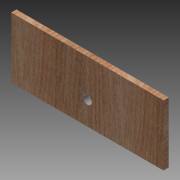
# Autodesk Inventor part: CNC-X-axis- foundation faces
Saved by Autodesk Inventor 2015 (Build 190159000, 159)
## iProperties
Created: 2015-03-20
Part Number: CNC-X-axis- foundation faces
Material: Generic
Document SubType Name: Modeling
Designer: Bangladesh
Density: 1 g/cm^3
Appearance: Default
Author: Bangladesh
Autodesk Inventor part; units mm, degrees
ref_plane "YZ Plane" through (0, 0, 0) normal (1, 0, 0) x (0, 1, 0)
ref_plane "XZ Plane" through (0, 0, 0) normal (0, 1, 0) x (-1, 0, 0)
ref_plane "XY Plane" through (0, 0, 0) normal (0, 0, 1) x (1, 0, 0)
sketch "Sketch1" plane through (0, 0, 0) normal (0, 0, 1) x (1, 0, 0)
  line L0 (-191, 76.2) -> (191, 76.2)
  line L1 (191, 76.2) -> (191, -76.2)
  line L2 (191, -76.2) -> (-191, -76.2)
  line L3 (-191, -76.2) -> (-191, 76.2)
  line L4 (-191, 76.2) -> (191, -76.2) construction
  line L5 (191, 76.2) -> (-191, -76.2) construction
  point P0 (0, 0)
  dimension "d0" = 152.4
  dimension "d1" = 382
  constraints: 12 end point, 2 midpoint, 2 parallel, 1 horizontal, 1 perpendicular
  measures "d0" distance of L0.end L1.end
  measures "d1" distance of L1.end L2.end
extrude "Extrusion1" add sketch "Sketch1" along normal mid plane 13
sketch "Sketch3" plane through (0, 0, 6.5) normal (0, 0, 1) x (1, 0, 0)
  circle A0 centre (15.76, -1.94) radius 0.8126
  circle A1 centre (-15.76, -1.94) radius 0.8126
  circle A2 centre (15.76, -33.46) radius 0.8126
  circle A3 centre (-15.76, -33.46) radius 0.8126
  line L0 (-15.76, -1.94) -> (15.76, -1.94)
  line L1 (15.76, -1.94) -> (15.76, -33.46)
  line L2 (15.76, -33.46) -> (-15.76, -33.46)
  line L3 (-15.76, -33.46) -> (-15.76, -1.94)
  line L4 (-15.76, -1.94) -> (15.76, -33.46) construction
  line L5 (15.76, -1.94) -> (-15.76, -33.46) construction
  line L6 (-191, -76.2) -> (191, -76.2) projected
  line L7 (-191, 76.2) -> (-191, -76.2) projected
  point P0 (0, 0)
  point P1 (0, -17.7)
  point P2 (0, -17.7)
  dimension "d5" = 31.52
  dimension "d6" = 31.52
  dimension "d7" = 58.5
  constraints: 12 end point, 4 centre point, 4 coincident, 4 midpoint, 2 parallel, 1 horizontal, 1 perpendicular, 1 vertical alignment
  measures "d5" distance of L0.end L1.end
  measures "d6" distance of L1.end L2.end
  measures "d7" distance from line of L6 point (0, -17.7)
hole "Hole1" at (15.76, -1.94, 6.5) at (-15.76, -1.94, 6.5) at (-15.76, -33.46, 6.5) at (15.76, -33.46, 6.5) direction (0, 0, -1) diameter 1.6252 end through all
sketch "Sketch4" plane through (0, 0, 6.5) normal (0, 0, 1) x (1, 0, 0)
  circle A0 centre (-15.76, -1.94) radius 0.8126 projected
  circle A1 centre (15.76, -33.46) radius 0.8126 projected
  circle A2 centre (0, -17.7) radius 11
  point P0 (0, 0)
  dimension "d18" = 22
  constraints: 1 centre point
  measures "d18" diameter of A2
hole "Hole2" at (0, -17.7, 6.5) direction (0, 0, -1) diameter 22 end through all
body "Solid1"
